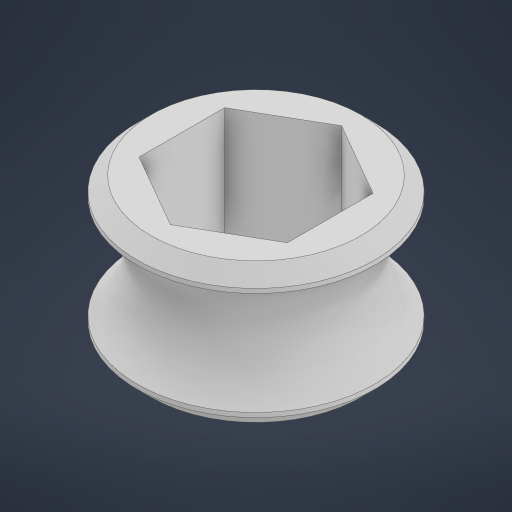
# Autodesk Inventor part: 5mm Hex Bearing Inside
Saved by Autodesk Inventor 2023 (Build 270158000, 158)
## iProperties
Created: 2022-10-15
Part Number: 5mm Hex Bearing Inside
Material: Generic
Document SubType Name: Modeling
Designer: izack
Density: 1 g/cm^3
Appearance: Default
Author: izack
## iProperties of the stored document 5mm Hex Bearing Inside_3DPrint.ipt
Part Number: 5mm Hex Bearing Inside_3DPrint
Material: Generic
Document SubType Name: Modeling
Designer: izack
Appearance: Default
Author: izack
Autodesk Inventor part; units mm, degrees
ref_plane "YZ Plane" through (0, 0, 0) normal (1, 0, 0) x (0, 1, 0)
ref_plane "XZ Plane" through (0, 0, 0) normal (0, 1, 0) x (-1, 0, 0)
ref_plane "XY Plane" through (0, 0, 0) normal (0, 0, 1) x (1, 0, 0)
sketch "Sketch1" plane through (0, 0, 0) normal (0, 1, 0) x (-1, 0, 0)
  line L0 (2.65, -1.53) -> (0, -3.06)
  line L1 (0, -3.06) -> (-2.65, -1.53)
  line L2 (-2.65, -1.53) -> (-2.65, 1.53)
  line L3 (-2.65, 1.53) -> (0, 3.06)
  line L4 (0, 3.06) -> (2.65, 1.53)
  line L5 (2.65, 1.53) -> (2.65, -1.53)
  circle A0 centre (0, 0) radius 3.5
  dimension "d1" = 5.3
  dimension "d2" = 7
  constraints: 12 end point, 2 coincident, 1 centre point, 13 other
  measures "d1" distance between parallel lines of L2 L5
  measures "d2" diameter of A0
extrude "Extrusion1" add sketch "Sketch1" along normal blind 5
sketch "Sketch2" plane through (0, 0, 0) normal (1, 0, 0) x (0, 1, 0)
  line L0 (0, -3.5) -> (5, -3.5) projected
  circle A0 centre (2.5, -5.75) radius 2.375
  line L1 (5, -3.5) -> (5, 3.5) projected
  line L2 (5, -3.5) -> (5, -4.25)
  line L3 (5, -4.25) -> (4.3414, -4.25)
  line L4 (0, -3.5) -> (0, 3.5) projected
  line L5 (0, -3.5) -> (0, -4.25)
  line L6 (0, -4.25) -> (0.6586, -4.25)
  line L7 (-1, 0) -> (6, 0) projected
  point P0 (0, 0)
  point P1 (1.7397, -3.5)
  point P2 (3.2603, -3.5)
  dimension "d5" = 4.75
  dimension "d6" = 2.25
  dimension "d7" = 0.75
  dimension "d8" = 0.75
  constraints: 8 end point, 2 point on circle, 2 point on line, 1 centre point, 1 perpendicular, 1 vertical
  measures "d5" diameter of A0
  measures "d6" distance from line of A0.centre L0
  measures "d7" distance of L0.end L2.end
  measures "d8" distance of L0.start L5.end
revolve "Revolution1" cut sketch "Sketch2" angle 360 about axis through (0, -10, 0) along (0, 1, 0) contours A0 L0 | L0 A0
revolve "Revolution2" add sketch "Sketch2" angle 360 about axis through (0, -10, 0) along (0, 1, 0) contours L0 A0 L6 L5 | L0 L2 L3 A0
chamfer "Chamfer1" distance 0.5 angle 45 2 edges at (0, 5, 4.25) (0, 0, 4.25)
ref_plane "Work Plane1" through (0, 2.5, 0) normal (0, 1, 0) x (1, 0, 0)
sketch "Sketch3" plane through (0, 0, 0) normal (0, -1, 0) x (1, 0, 0)
  line L0 (-2.65, -1.53) -> (0, -3.06) projected
  line L1 (-2.65, 1.53) -> (-2.65, -1.53) projected
  line L2 (0, 3.06) -> (-2.65, 1.53) projected
  line L3 (2.65, 1.53) -> (0, 3.06) projected
  line L4 (2.65, -1.53) -> (2.65, 1.53) projected
  line L5 (0, -3.06) -> (2.65, -1.53) projected
  circle A0 centre (0, 0) radius 3.75 projected
body "Solid1"
